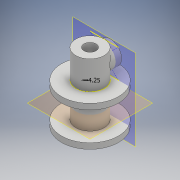
# Autodesk Inventor part: stationarySpindle
Saved by Autodesk Inventor 2018 (Build 220112000, 112)
## iProperties
Created: 2018-11-25
Part Number: stationarySpindle
Material: Generic
Document SubType Name: Modeling
Designer: Prakash
Density: 1 g/cm^3
Appearance: Default
Author: Prakash
Autodesk Inventor part; units mm, degrees
ref_plane "YZ Plane" through (0, 0, 0) normal (1, 0, 0) x (0, 1, 0)
ref_plane "XZ Plane" through (0, 0, 0) normal (0, 1, 0) x (-1, 0, 0)
ref_plane "XY Plane" through (0, 0, 0) normal (0, 0, 1) x (1, 0, 0)
sketch "Sketch1" plane through (0, 0, 0) normal (0, 0, 1) x (1, 0, 0)
  circle A0 centre (0, 0) radius 5
  circle A1 centre (0, 0) radius 10
  circle A2 centre (0, 0) radius 2.125
  dimension "d0" = 10
  dimension "d1" = 20
  dimension "d2" = 4.25
  constraints: 3 centre point, 3 coincident
  measures "d0" diameter of A0
  measures "d1" diameter of A1
  measures "d2" diameter of A2
extrude "Extrusion1" add sketch "Sketch1" against normal blind 10 contours A0 | A2
extrude "Extrusion2" add sketch "Sketch1" along normal blind 2 contours A0 | A1 | A2
sketch "Sketch2" plane through (0, 0, -10) normal (0, 0, -1) x (-1, 0, 0)
  circle A0 centre (0, 0) radius 10 projected
extrude "Extrusion3" add sketch "Sketch2" along normal blind 2
sketch "Sketch3" plane through (0, 0, 2) normal (0, 0, 1) x (1, 0, 0)
  circle A0 centre (0, 0) radius 5 projected
  circle A1 centre (0, 0) radius 2.125
  dimension "d9" = 4.25
  constraints: 1 centre point, 1 coincident
  measures "d9" diameter of A1
extrude "Extrusion4" add sketch "Sketch3" along normal blind 10
ref_plane "Work Plane1" through (0, 0, -5) normal (0, 0, 1) x (1, 0, 0)
sketch "Sketch4" plane through (0, 0, -5) normal (0, 0, 1) x (1, 0, 0)
  circle A0 centre (0, 0) radius 5 projected
  arc A1 (1.5, 4.7697) -> (-1.5, 4.7697) centre (0, 0) ccw
  line L0 (0, 0) -> (0, 5) construction
  line L1 (-1.5, 4.7697) -> (-1.5, 9.7697)
  line L2 (-1.5, 9.7697) -> (1.5, 9.7697)
  line L3 (1.5, 9.7697) -> (1.5, 4.7697)
  dimension "d12" = 5
  dimension "d13" = 3
  constraints: 8 end point, 5 point on circle, 3 vertical, 1 centre point, 1 concentric, 1 perpendicular, 1 other
  measures "d12" distance of L1.start L1.end
  measures "d13" distance of L1.end L2.end
extrude "Extrusion5" add sketch "Sketch4" along normal mid plane 3 contours A0 L1 L2 L3
ref_plane "Work Plane2" through (0, 5, 2) normal (0, 1, 0) x (-1, 0, 0)
sketch "Sketch5" plane through (0, 5, 2) normal (0, 1, 0) x (-1, 0, 0)
  line L0 (5, 10) -> (-5, 10) projected
  line L1 (-5, 0) -> (5, 0) projected
  line L2 (-5, 10) -> (5, 0) construction
  line L3 (5, 10) -> (-5, 0) construction
  point P0 (0, -2)
  point P1 (0, 5)
  constraints: 4 end point, 1 midpoint, 1 perpendicular
extrude "Extrusion6" cut sketch "Sketch3" against normal up to surface (14 mm away) contours A1
sketch "Sketch6" plane through (0, 5, 2) normal (0, 1, 0) x (-1, 0, 0)
  line L0 (5, 10) -> (-5, 0) construction
  line L1 (-5, 10) -> (5, 0) construction
  circle A0 centre (0, 5) radius 4
  point P0 (0, -2)
  dimension "d18" = 8
  constraints: 1 centre point, 1 coincident
  measures "d18" diameter of A0
extrude "Extrusion7" add sketch "Sketch6" against normal up to surface round surface about axis through (0, 0, 2) along (0, 0, 1) radius 5 far side no
extrude "Extrusion8" add sketch "Sketch6" along normal blind 2.125
sketch "Sketch7" plane through (0, 7.125, 7) normal (0, 1, 0) x (1, 0, 0)
  line L0 (5, -5) -> (-5, 5) construction
  line L1 (-5, -5) -> (5, 5) construction
  circle A0 centre (0, 0) radius 4 projected
  circle A1 centre (0, 0) radius 2.5275
  point P0 (0, 7)
  dimension "d23" = 5.055
  constraints: 1 centre point, 1 coincident
  measures "d23" diameter of A1
extrude "Extrusion9" cut sketch "Sketch7" against normal blind 3.81 contours A1
sketch "Sketch8" plane through (0, 7.125, 7) normal (0, 1, 0) x (1, 0, 0)
  line L0 (-5, -5) -> (5, 5) construction
  line L1 (5, -5) -> (-5, 5) construction
  circle A0 centre (0, 0) radius 2.6545
  point P0 (0, 7)
  dimension "d26" = 5.309
  constraints: 1 centre point, 1 coincident
  measures "d26" diameter of A0
loft "Loft1" cut profiles "Sketch8" section 1 edges at (-2.5275, 3.315, 7)
sketch "Sketch9" plane through (0, 3.315, 7) normal (0, 1, 0) x (1, 0, 0)
  line L0 (-5, -5) -> (5, 5) construction
  line L1 (5, -5) -> (-5, 5) construction
  circle A0 centre (0, 0) radius 1.8
  point P0 (0, 7)
  dimension "d31" = 3.6
  constraints: 1 centre point, 1 coincident
  measures "d31" diameter of A0
extrude "Extrusion10" cut sketch "Sketch9" against normal up to surface round surface about axis through (0, 0, 2) along (0, 0, 1) radius 2.125 far side no
body "Solid1"
